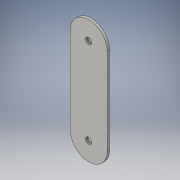
# Autodesk Inventor part: servo_arm
Saved by Autodesk Inventor 2016 (Build 200138000, 138)
## iProperties
Created: 2015-07-20
Part Number: servo_arm
Material: Generic
Document SubType Name: Modeling
Designer: chdsbd
Density: 1 g/cm^3
Appearance: Default
Author: chdsbd
Autodesk Inventor part; units mm, degrees
ref_plane "YZ Plane" through (0, 0, 0) normal (1, 0, 0) x (0, 1, 0)
ref_plane "XZ Plane" through (0, 0, 0) normal (0, 1, 0) x (-1, 0, 0)
ref_plane "XY Plane" through (0, 0, 0) normal (0, 0, 1) x (1, 0, 0)
sketch "Sketch1" plane through (0, 0, 0) normal (0, 0, 1) x (1, 0, 0)
  line L0 (0, 0) -> (0, 88.9) construction
  line L1 (19.05, 0) -> (19.05, 88.9)
  line L2 (-19.05, 88.9) -> (-19.05, 0)
  arc A0 (-19.05, 0) -> (19.05, 0) centre (0, 0) ccw
  arc A1 (19.05, 88.9) -> (-19.05, 88.9) centre (0, 88.9) ccw
  circle A2 centre (0, 88.9) radius 3.175
  circle A3 centre (0, 0) radius 3.175
  line L3 (-3.175, 0) -> (-5.715, 0)
  line L4 (0, -3.175) -> (0, -5.715)
  line L5 (3.175, 0) -> (5.715, 0)
  line L6 (0, 3.175) -> (0, 5.715)
  point P0 (0, 44.45)
  dimension "d5" = 6.35
  dimension "d0" = 88.9
  dimension "d1" = 38.1
  dimension "d2" = 6.35
  dimension "d9" = 2.54
  dimension "d12" = 360
  constraints: 16 end point, 4 point on circle, 4 tangent, 3 centre point, 2 coincident, 2 horizontal, 1 horizontal alignment, 1 midpoint, 1 parallel, 1 vertical, 15 other
  measures "d0" distance of L0.start L0.end
  measures "d1" distance between parallel lines of L2 L1
  measures "d2" diameter of A2
  measures "d9" distance of L3.start L3.end
extrude "Extrusion1" add sketch "Sketch1" along normal blind 2.54
body "Solid1"
